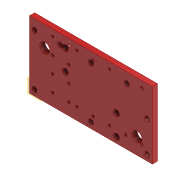
# Autodesk Inventor part: Motor mount to inside wall adapter
Saved by Autodesk Inventor 2020 (Build 240168000, 168)
## iProperties
Created: 2020-03-03
Part Number: Motor mount to inside wall adapter
Material: Generic
Document SubType Name: Modeling
Designer: ball
Density: 1 g/cm^3
Appearance: Default
Author: ball
Autodesk Inventor part; units mm, degrees
ref_plane "YZ Plane" through (0, 0, 0) normal (1, 0, 0) x (0, 1, 0)
ref_plane "XZ Plane" through (0, 0, 0) normal (0, 1, 0) x (-1, 0, 0)
ref_plane "XY Plane" through (0, 0, 0) normal (0, 0, 1) x (1, 0, 0)
ref_plane "Work Plane2" through (0, 0, 0) normal (0, 0, 1) x (1, 0, 0)
sketch "Sketch1" plane through (0, 0, 0) normal (0, 0, 1) x (1, 0, 0)
  line L0 (192, 96) -> (192, 48) construction
  line L1 (0, 96) -> (0, 48) construction
  line L2 (0, 0) -> (0, 48) construction
  line L3 (0, 0) -> (0, 96)
  line L4 (192, 96) -> (192, 0)
  circle A0 centre (184, 8) radius 2 construction
  circle A1 centre (8, 8) radius 2 construction
  circle A2 centre (8, 88) radius 2 construction
  circle A3 centre (184, 56) radius 2 construction
  arc A4 (98, 88) -> (94, 88) centre (96, 88) ccw construction
  arc A5 (94, 8) -> (98, 8) centre (96, 8) ccw construction
  circle A6 centre (184, 8) radius 2.2
  circle A7 centre (96, 8) radius 2.2
  circle A8 centre (8, 8) radius 2.2
  circle A9 centre (8, 88) radius 2.2
  circle A10 centre (96, 88) radius 2.2
  circle A11 centre (184, 56) radius 2.2
  circle A12 centre (152, 88) radius 2 construction
  circle A13 centre (152, 88) radius 2.2
  circle A14 centre (56, 88) radius 3.5 construction
  circle A15 centre (56, 56) radius 3.5 construction
  circle A16 centre (136, 8) radius 3.5 construction
  circle A17 centre (136, 40) radius 3.5 construction
  circle A18 centre (136, 8) radius 4.5
  circle A19 centre (136, 40) radius 4.5
  circle A20 centre (56, 88) radius 4.5
  circle A21 centre (56, 56) radius 4.5
  circle A22 centre (24, 72) radius 7.78 projected
  circle A23 centre (168, 24) radius 7.78 projected
  line L5 (0, 96) -> (0, 103.6708)
  line L6 (0, 103.6708) -> (192, 103.6708)
  line L7 (192, 103.6708) -> (192, 96)
  line L8 (0, 0) -> (0, -1.2954)
  line L9 (0, -1.2954) -> (192, -1.2954)
  line L10 (192, -1.2954) -> (192, 0)
  dimension "d0" = 4.4
  dimension "d1" = 4.4
  dimension "d2" = 4.4
  dimension "d3" = 4.4
  dimension "d4" = 4.4
  dimension "d5" = 4.4
  dimension "d6" = 4.4
  dimension "d7" = 9
  dimension "d8" = 9
  dimension "d9" = 9
  dimension "d10" = 9
  constraints: 16 end point, 11 centre point, 11 coincident, 3 parallel, 1 point on line
  measures "d0" diameter of A6
  measures "d1" diameter of A7
  measures "d2" diameter of A8
  measures "d3" diameter of A9
  measures "d4" diameter of A10
  measures "d5" diameter of A11
  measures "d6" diameter of A13
  measures "d7" diameter of A18
  measures "d8" diameter of A19
  measures "d9" diameter of A20
  measures "d10" diameter of A21
extrude "Extrusion1" add sketch "Sketch1" along normal blind 8
sketch "Sketch2" plane through (0, 0, 8) normal (0, 0, 1) x (1, 0, 0)
  circle A0 centre (184, 8) radius 2.2 construction
  circle A1 centre (184, 8) radius 4.115 construction
  line L0 (184, 12.115) -> (187.5637, 10.0575)
  line L1 (187.5637, 10.0575) -> (187.5637, 5.9425)
  line L2 (187.5637, 5.9425) -> (184, 3.885)
  line L3 (184, 3.885) -> (180.4363, 5.9425)
  line L4 (180.4363, 5.9425) -> (180.4363, 10.0575)
  line L5 (180.4363, 10.0575) -> (184, 12.115)
  circle A2 centre (96, 8) radius 2.2 construction
  circle A3 centre (96, 8) radius 4.115 construction
  circle A4 centre (8, 8) radius 2.2 construction
  circle A5 centre (8, 8) radius 4.115 construction
  circle A6 centre (8, 88) radius 2.2 construction
  circle A7 centre (8, 88) radius 4.115 construction
  circle A8 centre (96, 88) radius 2.2 construction
  circle A9 centre (96, 88) radius 4.115 construction
  circle A10 centre (184, 56) radius 2.2 construction
  circle A11 centre (184, 56) radius 4.115 construction
  line L6 (184, 60.115) -> (187.5637, 58.0575)
  line L7 (187.5637, 58.0575) -> (187.5637, 53.9425)
  line L8 (187.5637, 53.9425) -> (184, 51.885)
  line L9 (184, 51.885) -> (180.4363, 53.9425)
  line L10 (180.4363, 53.9425) -> (180.4363, 58.0575)
  line L11 (180.4363, 58.0575) -> (184, 60.115)
  line L12 (96, 92.115) -> (99.5637, 90.0575)
  line L13 (99.5637, 90.0575) -> (99.5637, 85.9425)
  line L14 (99.5637, 85.9425) -> (96, 83.885)
  line L15 (96, 83.885) -> (92.4363, 85.9425)
  line L16 (92.4363, 85.9425) -> (92.4363, 90.0575)
  line L17 (92.4363, 90.0575) -> (96, 92.115)
  line L18 (8, 92.115) -> (11.5637, 90.0575)
  line L19 (11.5637, 90.0575) -> (11.5637, 85.9425)
  line L20 (11.5637, 85.9425) -> (8, 83.885)
  line L21 (8, 83.885) -> (4.4363, 85.9425)
  line L22 (4.4363, 85.9425) -> (4.4363, 90.0575)
  line L23 (4.4363, 90.0575) -> (8, 92.115)
  line L24 (8, 12.115) -> (11.5637, 10.0575)
  line L25 (11.5637, 10.0575) -> (11.5637, 5.9425)
  line L26 (11.5637, 5.9425) -> (8, 3.885)
  line L27 (8, 3.885) -> (4.4363, 5.9425)
  line L28 (4.4363, 5.9425) -> (4.4363, 10.0575)
  line L29 (4.4363, 10.0575) -> (8, 12.115)
  line L30 (96, 12.115) -> (99.5637, 10.0575)
  line L31 (99.5637, 10.0575) -> (99.5637, 5.9425)
  line L32 (99.5637, 5.9425) -> (96, 3.885)
  line L33 (96, 3.885) -> (92.4363, 5.9425)
  line L34 (92.4363, 5.9425) -> (92.4363, 10.0575)
  line L35 (92.4363, 10.0575) -> (96, 12.115)
  circle A12 centre (152, 88) radius 2.2 construction
  circle A13 centre (152, 88) radius 4.115 construction
  line L36 (152, 92.115) -> (155.5637, 90.0575)
  line L37 (155.5637, 90.0575) -> (155.5637, 85.9425)
  line L38 (155.5637, 85.9425) -> (152, 83.885)
  line L39 (152, 83.885) -> (148.4363, 85.9425)
  line L40 (148.4363, 85.9425) -> (148.4363, 90.0575)
  line L41 (148.4363, 90.0575) -> (152, 92.115)
  point P0 (0, 0)
  dimension "d13" = 8.23
  dimension "d16" = 8.23
  dimension "d17" = 8.23
  dimension "d18" = 8.23
  dimension "d19" = 8.23
  dimension "d20" = 8.23
  dimension "d66" = 8.23
  constraints: 84 end point, 14 coincident, 7 vertical alignment, 105 other
extrude "Nut Well 4mm" cut sketch "Sketch2" against normal blind 5.5
sketch "Sketch3" plane through (0, 0, 0) normal (0, 0, -1) x (-1, 0, 0)
  circle A0 centre (-36.0247, 17.3171) radius 1.9304 construction
  circle A1 centre (-61.4247, 17.3171) radius 1.9304 construction
  circle A2 centre (-61.4247, 42.7171) radius 1.9304 construction
  circle A3 centre (-36.0247, 42.7171) radius 1.9304 construction
  circle A4 centre (-36.0247, 68.1171) radius 1.9304 construction
  circle A5 centre (-61.4247, 68.1171) radius 1.9304 construction
  circle A6 centre (-61.4247, 93.5171) radius 1.9304 construction
  circle A7 centre (-36.0247, 93.5171) radius 1.9304 construction
  circle A8 centre (-74.1247, 93.5171) radius 1.9304 construction
  circle A9 centre (-99.5247, 93.5171) radius 1.9304 construction
  circle A10 centre (-124.9247, 93.5171) radius 1.9304 construction
  circle A11 centre (-99.5247, 68.1171) radius 1.9304 construction
  circle A12 centre (-74.1247, 68.1171) radius 1.9304 construction
  circle A13 centre (-74.1247, 42.7171) radius 1.9304 construction
  circle A14 centre (-99.5247, 42.7171) radius 1.9304 construction
  circle A15 centre (-124.9247, 42.7171) radius 1.9304 construction
  line L0 (-192, -1.2954) -> (-192, 103.6708) construction
  line L1 (0, -1.2954) -> (-192, -1.2954) construction
  line L2 (0, 103.6708) -> (0, -1.2954) construction
  line L3 (-192, 103.6708) -> (0, 103.6708) construction
  circle A16 centre (-168, 24) radius 7.78 construction
  circle A17 centre (-56, 56) radius 4.5 construction
  circle A18 centre (-136, 40) radius 4.5 construction
  circle A19 centre (-184, 8) radius 2.2 construction
  circle A20 centre (-96, 8) radius 2.2 construction
  circle A21 centre (-8, 8) radius 2.2 construction
  circle A22 centre (-8, 88) radius 2.2 construction
  circle A23 centre (-96, 88) radius 2.2 construction
  circle A24 centre (-184, 56) radius 2.2 construction
  circle A25 centre (-152, 88) radius 2.2 construction
  circle A26 centre (-136, 8) radius 4.5 construction
  circle A27 centre (-56, 88) radius 4.5 construction
  circle A28 centre (-24, 72) radius 7.78 construction
  circle A29 centre (-124.9247, 68.1171) radius 1.9304 construction
  circle A30 centre (-150.3247, 68.1171) radius 1.9304 construction
  circle A31 centre (-175.7247, 68.1171) radius 1.9304 construction
  circle A32 centre (-150.3247, 42.7171) radius 1.9304 construction
  circle A33 centre (-175.7247, 42.7171) radius 1.9304 construction
  circle A34 centre (-175.7247, 17.3171) radius 1.9304 construction
  circle A35 centre (-150.3247, 17.3171) radius 1.9304 construction
  circle A36 centre (-124.9247, 17.3171) radius 1.9304 construction
  circle A37 centre (-99.5247, 17.3171) radius 1.9304 construction
  circle A38 centre (-74.1247, 17.3171) radius 1.9304 construction
  circle A39 centre (-175.7247, 93.5171) radius 1.9304 construction
  circle A40 centre (-150.3247, 93.5171) radius 1.9304 construction
  circle A41 centre (-36.0247, 17.3171) radius 1.9304
  circle A42 centre (-36.0247, 42.7171) radius 1.9304
  circle A43 centre (-36.0247, 68.1171) radius 1.9304
  circle A44 centre (-36.0247, 93.5171) radius 1.9304
  circle A45 centre (-61.4247, 68.1171) radius 1.9304
  circle A46 centre (-61.4247, 42.7171) radius 1.9304
  circle A47 centre (-61.4247, 17.3171) radius 1.9304
  circle A48 centre (-74.1247, 93.5171) radius 1.9304
  circle A49 centre (-74.1247, 17.3171) radius 1.9304
  circle A50 centre (-99.5247, 17.3171) radius 1.9304
  circle A51 centre (-124.9247, 17.3171) radius 1.9304
  circle A52 centre (-150.3247, 17.3171) radius 1.9304
  circle A53 centre (-175.7247, 17.3171) radius 1.9304
  circle A54 centre (-175.7247, 93.5171) radius 1.9304
  circle A55 centre (-124.9247, 93.5171) radius 1.9304
  circle A56 centre (-99.5247, 93.5171) radius 1.9304
  circle A57 centre (-56, 88) radius 3.5052 construction
  circle A58 centre (-61.4247, 93.5171) radius 1.9304
  point P0 (0, 0)
  dimension "SixClearanceHole" = 3.8608
  dimension "d26" = 3.8608
  dimension "d27" = 3.8608
  dimension "d28" = 3.8608
  dimension "d29" = 3.8608
  dimension "d30" = 3.8608
  dimension "d31" = 3.8608
  dimension "d32" = 3.8608
  dimension "d33" = 3.8608
  dimension "d34" = 3.8608
  dimension "d35" = 3.8608
  dimension "d36" = 3.8608
  dimension "d37" = 3.8608
  dimension "d38" = 3.8608
  dimension "d39" = 3.8608
  dimension "d40" = 3.8608
  dimension "d41" = 7.0104
  dimension "d42" = 3.8608
  constraints: 18 centre point, 18 coincident
  measures "SixClearanceHole" diameter of A41
  measures "d26" diameter of A42
  measures "d27" diameter of A43
  measures "d28" diameter of A44
  measures "d29" diameter of A45
  measures "d30" diameter of A46
  measures "d31" diameter of A47
  measures "d32" diameter of A48
  measures "d33" diameter of A49
  measures "d34" diameter of A50
  measures "d35" diameter of A51
  measures "d36" diameter of A52
  measures "d37" diameter of A53
  measures "d38" diameter of A54
  measures "d39" diameter of A55
  measures "d40" diameter of A56
  measures "d41" diameter of A57
  measures "d42" diameter of A58
extrude "Extrusion3" cut sketch "Sketch3" against normal through all
sketch "Sketch4" plane through (0, 0, 0) normal (0, 0, -1) x (-1, 0, 0)
  circle A0 centre (-36.0247, 17.3171) radius 1.9304 construction
  circle A1 centre (-36.0247, 17.3171) radius 4.6609 construction
  line L0 (-36.0247, 21.978) -> (-31.9883, 19.6475)
  line L1 (-31.9883, 19.6475) -> (-31.9883, 14.9866)
  line L2 (-31.9883, 14.9866) -> (-36.0247, 12.6562)
  line L3 (-36.0247, 12.6562) -> (-40.0612, 14.9866)
  line L4 (-40.0612, 14.9866) -> (-40.0612, 19.6475)
  line L5 (-40.0612, 19.6475) -> (-36.0247, 21.978)
  circle A2 centre (-36.0247, 42.7171) radius 1.9304 construction
  circle A3 centre (-36.0247, 68.1171) radius 1.9304 construction
  circle A4 centre (-36.0247, 93.5171) radius 1.9304 construction
  circle A5 centre (-74.1247, 93.5171) radius 1.9304 construction
  circle A6 centre (-124.9247, 93.5171) radius 1.9304 construction
  circle A7 centre (-175.7247, 93.5171) radius 1.9304 construction
  circle A8 centre (-184, 8) radius 2.2 construction
  circle A9 centre (-61.4247, 68.1171) radius 1.9304 construction
  circle A10 centre (-61.4247, 42.7171) radius 1.9304 construction
  circle A11 centre (-61.4247, 17.3171) radius 1.9304 construction
  circle A12 centre (-36.0247, 42.7171) radius 4.6609 construction
  line L6 (-36.0247, 47.378) -> (-31.9883, 45.0475)
  line L7 (-31.9883, 45.0475) -> (-31.9883, 40.3866)
  line L8 (-31.9883, 40.3866) -> (-36.0247, 38.0562)
  line L9 (-36.0247, 38.0562) -> (-40.0612, 40.3866)
  line L10 (-40.0612, 40.3866) -> (-40.0612, 45.0475)
  line L11 (-40.0612, 45.0475) -> (-36.0247, 47.378)
  circle A13 centre (-36.0247, 68.1171) radius 4.6609 construction
  line L12 (-36.0247, 72.778) -> (-31.9883, 70.4475)
  line L13 (-31.9883, 70.4475) -> (-31.9883, 65.7866)
  line L14 (-31.9883, 65.7866) -> (-36.0247, 63.4562)
  line L15 (-36.0247, 63.4562) -> (-40.0612, 65.7866)
  line L16 (-40.0612, 65.7866) -> (-40.0612, 70.4475)
  line L17 (-40.0612, 70.4475) -> (-36.0247, 72.778)
  circle A14 centre (-36.0247, 93.5171) radius 4.6609 construction
  line L18 (-36.0247, 98.178) -> (-31.9883, 95.8475)
  line L19 (-31.9883, 95.8475) -> (-31.9883, 91.1866)
  line L20 (-31.9883, 91.1866) -> (-36.0247, 88.8562)
  line L21 (-36.0247, 88.8562) -> (-40.0612, 91.1866)
  line L22 (-40.0612, 91.1866) -> (-40.0612, 95.8475)
  line L23 (-40.0612, 95.8475) -> (-36.0247, 98.178)
  circle A15 centre (-61.4247, 68.1171) radius 4.6609 construction
  line L24 (-61.4247, 72.778) -> (-57.3883, 70.4475)
  line L25 (-57.3883, 70.4475) -> (-57.3883, 65.7866)
  line L26 (-57.3883, 65.7866) -> (-61.4247, 63.4562)
  line L27 (-61.4247, 63.4562) -> (-65.4612, 65.7866)
  line L28 (-65.4612, 65.7866) -> (-65.4612, 70.4475)
  line L29 (-65.4612, 70.4475) -> (-61.4247, 72.778)
  circle A16 centre (-61.4247, 42.7171) radius 4.6609 construction
  line L30 (-61.4247, 47.378) -> (-57.3883, 45.0475)
  line L31 (-57.3883, 45.0475) -> (-57.3883, 40.3866)
  line L32 (-57.3883, 40.3866) -> (-61.4247, 38.0562)
  line L33 (-61.4247, 38.0562) -> (-65.4612, 40.3866)
  line L34 (-65.4612, 40.3866) -> (-65.4612, 45.0475)
  line L35 (-65.4612, 45.0475) -> (-61.4247, 47.378)
  circle A17 centre (-61.4247, 17.3171) radius 4.6609 construction
  line L36 (-61.4247, 21.978) -> (-57.3883, 19.6475)
  line L37 (-57.3883, 19.6475) -> (-57.3883, 14.9866)
  line L38 (-57.3883, 14.9866) -> (-61.4247, 12.6562)
  line L39 (-61.4247, 12.6562) -> (-65.4612, 14.9866)
  line L40 (-65.4612, 14.9866) -> (-65.4612, 19.6475)
  line L41 (-65.4612, 19.6475) -> (-61.4247, 21.978)
  circle A18 centre (-61.4247, 93.5171) radius 1.9304 construction
  circle A19 centre (-61.4247, 93.5171) radius 4.6609 construction
  circle A20 centre (-74.1247, 93.5171) radius 4.6609 construction
  circle A21 centre (-124.9247, 93.5171) radius 4.6609 construction
  circle A22 centre (-175.7247, 93.5171) radius 4.6609 construction
  line L42 (-61.4247, 98.178) -> (-57.3883, 95.8475)
  line L43 (-57.3883, 95.8475) -> (-57.3883, 91.1866)
  line L44 (-57.3883, 91.1866) -> (-61.4247, 88.8562)
  line L45 (-61.4247, 88.8562) -> (-65.4612, 91.1866)
  line L46 (-65.4612, 91.1866) -> (-65.4612, 95.8475)
  line L47 (-65.4612, 95.8475) -> (-61.4247, 98.178)
  line L48 (-74.1247, 98.178) -> (-70.0883, 95.8475)
  line L49 (-70.0883, 95.8475) -> (-70.0883, 91.1866)
  line L50 (-70.0883, 91.1866) -> (-74.1247, 88.8562)
  line L51 (-74.1247, 88.8562) -> (-78.1612, 91.1866)
  line L52 (-78.1612, 91.1866) -> (-78.1612, 95.8475)
  line L53 (-78.1612, 95.8475) -> (-74.1247, 98.178)
  line L54 (-124.9247, 98.178) -> (-120.8883, 95.8475)
  line L55 (-120.8883, 95.8475) -> (-120.8883, 91.1866)
  line L56 (-120.8883, 91.1866) -> (-124.9247, 88.8562)
  line L57 (-124.9247, 88.8562) -> (-128.9612, 91.1866)
  line L58 (-128.9612, 91.1866) -> (-128.9612, 95.8475)
  line L59 (-128.9612, 95.8475) -> (-124.9247, 98.178)
  line L60 (-175.7247, 98.178) -> (-171.6883, 95.8475)
  line L61 (-171.6883, 95.8475) -> (-171.6883, 91.1866)
  line L62 (-171.6883, 91.1866) -> (-175.7247, 88.8562)
  line L63 (-175.7247, 88.8562) -> (-179.7612, 91.1866)
  line L64 (-179.7612, 91.1866) -> (-179.7612, 95.8475)
  line L65 (-179.7612, 95.8475) -> (-175.7247, 98.178)
  point P0 (0, 0)
  point P1 (-99.5247, 93.5171)
  dimension "d45" = 9.3218
  dimension "d49" = 9.3218
  dimension "d50" = 9.3218
  dimension "d51" = 9.3218
  dimension "d52" = 9.3218
  dimension "d53" = 9.3218
  dimension "d73" = 9.3218
  dimension "d74" = 9.3218
  dimension "d76" = 9.3218
  dimension "d77" = 9.3218
  dimension "SixNutWell" = 9.3218
  constraints: 132 end point, 11 vertical alignment, 10 coincident, 165 other
extrude "Lift receiver nut wells thick plastic" cut sketch "Sketch4" against normal blind 6.7564
sketch "Sketch5" plane through (0, 0, 0) normal (0, 0, -1) x (-1, 0, 0)
  circle A0 centre (-74.1247, 17.3171) radius 1.9304 construction
  circle A1 centre (-74.1247, 17.3171) radius 4.6609 construction
  circle A2 centre (-99.5247, 17.3171) radius 1.9304 construction
  circle A3 centre (-99.5247, 17.3171) radius 4.6609 construction
  circle A4 centre (-124.9247, 17.3171) radius 1.9304 construction
  circle A5 centre (-124.9247, 17.3171) radius 4.6609 construction
  circle A6 centre (-150.3247, 17.3171) radius 1.9304 construction
  circle A7 centre (-150.3247, 17.3171) radius 4.6609 construction
  line L0 (-74.1247, 21.978) -> (-70.0883, 19.6475)
  line L1 (-70.0883, 19.6475) -> (-70.0883, 14.9866)
  line L2 (-70.0883, 14.9866) -> (-74.1247, 12.6562)
  line L3 (-74.1247, 12.6562) -> (-78.1612, 14.9866)
  line L4 (-78.1612, 14.9866) -> (-78.1612, 19.6475)
  line L5 (-78.1612, 19.6475) -> (-74.1247, 21.978)
  line L6 (-99.5247, 21.978) -> (-95.4883, 19.6475)
  line L7 (-95.4883, 19.6475) -> (-95.4883, 14.9866)
  line L8 (-95.4883, 14.9866) -> (-99.5247, 12.6562)
  line L9 (-99.5247, 12.6562) -> (-103.5612, 14.9866)
  line L10 (-103.5612, 14.9866) -> (-103.5612, 19.6475)
  line L11 (-103.5612, 19.6475) -> (-99.5247, 21.978)
  line L12 (-124.9247, 21.978) -> (-120.8883, 19.6475)
  line L13 (-120.8883, 19.6475) -> (-120.8883, 14.9866)
  line L14 (-120.8883, 14.9866) -> (-124.9247, 12.6562)
  line L15 (-124.9247, 12.6562) -> (-128.9612, 14.9866)
  line L16 (-128.9612, 14.9866) -> (-128.9612, 19.6475)
  line L17 (-128.9612, 19.6475) -> (-124.9247, 21.978)
  line L18 (-150.3247, 21.978) -> (-146.2883, 19.6475)
  line L19 (-146.2883, 19.6475) -> (-146.2883, 14.9866)
  line L20 (-146.2883, 14.9866) -> (-150.3247, 12.6562)
  line L21 (-150.3247, 12.6562) -> (-154.3612, 14.9866)
  line L22 (-154.3612, 14.9866) -> (-154.3612, 19.6475)
  line L23 (-154.3612, 19.6475) -> (-150.3247, 21.978)
  point P0 (0, 0)
  dimension "d78" = 9.3218
  dimension "d79" = 9.3218
  dimension "d80" = 9.3218
  dimension "d81" = 9.3218
  constraints: 48 end point, 9 coincident, 4 vertical alignment, 60 other
extrude "Lift receiver nut wells thin plastic" cut sketch "Sketch5" against normal blind 6.9088
sketch "Sketch6" plane through (0, 0, 0) normal (0, 0, -1) x (-1, 0, 0)
  line L0 (-24.7886, 9.4478) -> (-24.7886, 4.073)
  line L1 (-24.7886, 4.073) -> (-22.7434, 4.073)
  line L2 (-22.7434, 4.073) -> (-22.7434, 3.3518)
  line L3 (-22.7434, 3.3518) -> (-27.6439, 3.3518)
  line L4 (-27.6439, 3.3518) -> (-27.6439, 4.073)
  line L5 (-27.6439, 4.073) -> (-25.5988, 4.073)
  line L6 (-25.5988, 4.073) -> (-25.5988, 9.4478)
  line L7 (-25.5988, 9.4478) -> (-24.7886, 9.4478)
  spline S0 degree 2 poles (-32.5741, 4.0483) (-32.9199, 4.4534) (-33.3052, 5.639) (-33.3052, 6.3998) knots 0 0 0 1 2 2 2
  spline S1 degree 2 poles (-33.3052, 6.3998) (-33.3052, 7.1408) (-32.9298, 8.3412) (-32.5741, 8.7463) knots 0 0 0 1 2 2 2
  spline S2 degree 2 poles (-32.5741, 8.7463) (-32.1987, 9.1711) (-31.2057, 9.5762) (-30.608, 9.5762) knots 0 0 0 1 2 2 2
  spline S3 degree 2 poles (-30.608, 9.5762) (-29.9905, 9.5762) (-29.0024, 9.1563) (-28.6418, 8.7463) knots 0 0 0 1 2 2 2
  spline S4 degree 2 poles (-28.6418, 8.7463) (-28.2911, 8.3412) (-27.9156, 7.1507) (-27.9156, 6.3998) knots 0 0 0 1 2 2 2
  spline S5 degree 2 poles (-27.9156, 6.3998) (-27.9156, 5.6341) (-28.296, 4.4682) (-28.6468, 4.0483) knots 0 0 0 1 2 2 2
  spline S6 degree 2 poles (-28.6468, 4.0483) (-29.0024, 3.6432) (-29.9954, 3.2233) (-30.608, 3.2233) knots 0 0 0 1 2 2 2
  spline S7 degree 2 poles (-30.608, 3.2233) (-31.2304, 3.2233) (-32.2283, 3.6581) (-32.5741, 4.0483) knots 0 0 0 1 2 2 2
  spline S8 degree 2 poles (-32.4605, 6.3998) (-32.4605, 5.7971) (-32.1987, 4.8634) (-31.9615, 4.5571) knots 0 0 0 1 2 2 2
  spline S9 degree 2 poles (-31.9615, 4.5571) (-31.7195, 4.241) (-31.0377, 3.9248) (-30.6129, 3.9248) knots 0 0 0 1 2 2 2
  spline S10 degree 2 poles (-30.6129, 3.9248) (-30.1732, 3.9248) (-29.5113, 4.2311) (-29.2593, 4.5571) knots 0 0 0 1 2 2 2
  spline S11 degree 2 poles (-29.2593, 4.5571) (-29.0173, 4.8684) (-28.7604, 5.807) (-28.7604, 6.3998) knots 0 0 0 1 2 2 2
  spline S12 degree 2 poles (-28.7604, 6.3998) (-28.7604, 7.6002) (-29.7682, 8.8747) (-30.6129, 8.8747) knots 0 0 0 1 2 2 2
  spline S13 degree 2 poles (-30.6129, 8.8747) (-31.4576, 8.8747) (-32.4605, 7.6002) (-32.4605, 6.3998) knots 0 0 0 1 2 2 2
  spline S14 degree 2 poles (-38.0476, 5.1895) (-38.0476, 5.5847) (-37.7661, 6.296) (-37.5141, 6.543) knots 0 0 0 1 2 2 2
  spline S15 degree 2 poles (-37.5141, 6.543) (-37.198, 6.8543) (-36.3433, 7.1754) (-35.6913, 7.1754) knots 0 0 0 1 2 2 2
  line L8 (-35.6913, 7.1754) -> (-35.0046, 7.1754)
  line L9 (-35.0046, 7.1754) -> (-35.0046, 9.4478)
  line L10 (-35.0046, 9.4478) -> (-34.1944, 9.4478)
  line L11 (-34.1944, 9.4478) -> (-34.1944, 3.3518)
  line L12 (-34.1944, 3.3518) -> (-35.7258, 3.3518)
  spline S16 degree 2 poles (-35.7258, 3.3518) (-36.2692, 3.3518) (-37.03, 3.5296) (-37.3215, 3.7322) knots 0 0 0 1 2 2 2
  spline S17 degree 2 poles (-37.3215, 3.7322) (-37.6623, 3.9643) (-38.0476, 4.6806) (-38.0476, 5.1895) knots 0 0 0 1 2 2 2
  spline S18 degree 2 poles (-37.2029, 5.2142) (-37.2029, 4.898) (-36.9855, 4.4336) (-36.7632, 4.2854) knots 0 0 0 1 2 2 2
  spline S19 degree 2 poles (-36.7632, 4.2854) (-36.5706, 4.157) (-36.0568, 4.0533) (-35.6764, 4.0533) knots 0 0 0 1 2 2 2
  line L13 (-35.6764, 4.0533) -> (-35.0046, 4.0533)
  line L14 (-35.0046, 4.0533) -> (-35.0046, 6.4838)
  line L15 (-35.0046, 6.4838) -> (-35.5579, 6.4838)
  spline S20 degree 2 poles (-35.5579, 6.4838) (-36.0519, 6.4838) (-36.6595, 6.3257) (-36.8571, 6.1182) knots 0 0 0 1 2 2 2
  spline S21 degree 2 poles (-36.8571, 6.1182) (-37.0399, 5.9354) (-37.2029, 5.5056) (-37.2029, 5.2142) knots 0 0 0 1 2 2 2
  line L16 (-78.4457, 43.6737) -> (-78.4457, 38.2989)
  line L17 (-78.4457, 38.2989) -> (-76.4006, 38.2989)
  line L18 (-76.4006, 38.2989) -> (-76.4006, 37.5777)
  line L19 (-76.4006, 37.5777) -> (-81.3011, 37.5777)
  line L20 (-81.3011, 37.5777) -> (-81.3011, 38.2989)
  line L21 (-81.3011, 38.2989) -> (-79.2559, 38.2989)
  line L22 (-79.2559, 38.2989) -> (-79.2559, 43.6737)
  line L23 (-79.2559, 43.6737) -> (-78.4457, 43.6737)
  line L24 (-86.3448, 43.6737) -> (-85.5347, 43.6737)
  line L25 (-85.5347, 43.6737) -> (-85.5347, 40.6899)
  line L26 (-85.5347, 40.6899) -> (-82.7287, 40.6899)
  line L27 (-82.7287, 40.6899) -> (-82.7287, 43.6737)
  line L28 (-82.7287, 43.6737) -> (-81.9186, 43.6737)
  line L29 (-81.9186, 43.6737) -> (-81.9186, 37.5777)
  line L30 (-81.9186, 37.5777) -> (-82.7287, 37.5777)
  line L31 (-82.7287, 37.5777) -> (-82.7287, 39.9686)
  line L32 (-82.7287, 39.9686) -> (-85.5347, 39.9686)
  line L33 (-85.5347, 39.9686) -> (-85.5347, 37.5777)
  line L34 (-85.5347, 37.5777) -> (-86.3448, 37.5777)
  line L35 (-86.3448, 37.5777) -> (-86.3448, 43.6737)
  line L36 (-89.7041, 43.6737) -> (-87.3427, 43.6737)
  line L37 (-87.3427, 43.6737) -> (-87.3427, 43.0512)
  line L38 (-87.3427, 43.0512) -> (-88.1183, 43.0512)
  line L39 (-88.1183, 43.0512) -> (-88.1183, 38.2001)
  line L40 (-88.1183, 38.2001) -> (-87.3427, 38.2001)
  line L41 (-87.3427, 38.2001) -> (-87.3427, 37.5777)
  line L42 (-87.3427, 37.5777) -> (-89.7041, 37.5777)
  line L43 (-89.7041, 37.5777) -> (-89.7041, 38.2001)
  line L44 (-89.7041, 38.2001) -> (-88.9285, 38.2001)
  line L45 (-88.9285, 38.2001) -> (-88.9285, 43.0512)
  line L46 (-88.9285, 43.0512) -> (-89.7041, 43.0512)
  line L47 (-89.7041, 43.0512) -> (-89.7041, 43.6737)
  spline S22 degree 2 poles (-92.4063, 43.7824) (-91.7443, 43.7824) (-90.8156, 43.5057) (-90.4055, 43.3081) knots 0 0 0 1 2 2 2
  line L48 (-90.4055, 43.3081) -> (-90.4055, 42.2905)
  line L49 (-90.4055, 42.2905) -> (-90.4648, 42.2905)
  spline S23 degree 2 poles (-90.4648, 42.2905) (-90.865, 42.6659) (-91.8777, 43.0809) (-92.347, 43.0809) knots 0 0 0 1 2 2 2
  spline S24 degree 2 poles (-92.347, 43.0809) (-93.0188, 43.0809) (-93.7055, 42.5226) (-93.7055, 42.0632) knots 0 0 0 1 2 2 2
  spline S25 degree 2 poles (-93.7055, 42.0632) (-93.7055, 41.6977) (-93.3449, 41.2432) (-92.9546, 41.1296) knots 0 0 0 1 2 2 2
  spline S26 degree 2 poles (-92.9546, 41.1296) (-92.673, 41.0505) (-92.2037, 40.9418) (-91.853, 40.8529) knots 0 0 0 1 2 2 2
  spline S27 degree 2 poles (-91.853, 40.8529) (-91.5368, 40.7689) (-91.0379, 40.517) (-90.8452, 40.3144) knots 0 0 0 1 2 2 2
  spline S28 degree 2 poles (-90.8452, 40.3144) (-90.6575, 40.1119) (-90.45, 39.5685) (-90.45, 39.2128) knots 0 0 0 1 2 2 2
  spline S29 degree 2 poles (-90.45, 39.2128) (-90.45, 38.4718) (-91.606, 37.469) (-92.5001, 37.469) knots 0 0 0 1 2 2 2
  spline S30 degree 2 poles (-92.5001, 37.469) (-93.0139, 37.469) (-93.9229, 37.6715) (-94.3131, 37.8642) knots 0 0 0 1 2 2 2
  line L50 (-94.3131, 37.8642) -> (-94.3131, 38.8324)
  line L51 (-94.3131, 38.8324) -> (-94.2538, 38.8324)
  spline S31 degree 2 poles (-94.2538, 38.8324) (-93.9624, 38.5657) (-93.0534, 38.1705) (-92.5545, 38.1705) knots 0 0 0 1 2 2 2
  spline S32 degree 2 poles (-92.5545, 38.1705) (-91.9913, 38.1705) (-91.2948, 38.6991) (-91.2948, 39.1288) knots 0 0 0 1 2 2 2
  spline S33 degree 2 poles (-91.2948, 39.1288) (-91.2948, 39.5142) (-91.7048, 39.9736) (-92.0901, 40.0773) knots 0 0 0 1 2 2 2
  spline S34 degree 2 poles (-92.0901, 40.0773) (-92.347, 40.1465) (-93.0929, 40.3243) (-93.3399, 40.3984) knots 0 0 0 1 2 2 2
  spline S35 degree 2 poles (-93.3399, 40.3984) (-93.9673, 40.5911) (-94.5502, 41.3667) (-94.5502, 41.9348) knots 0 0 0 1 2 2 2
  spline S36 degree 2 poles (-94.5502, 41.9348) (-94.5502, 42.2954) (-94.2588, 42.987) (-93.997, 43.2291) knots 0 0 0 1 2 2 2
  spline S37 degree 2 poles (-93.997, 43.2291) (-93.7055, 43.4958) (-92.9645, 43.7824) (-92.4063, 43.7824) knots 0 0 0 1 2 2 2
  spline S38 degree 2 poles (-99.6928, 43.7824) (-99.0308, 43.7824) (-98.1021, 43.5057) (-97.6921, 43.3081) knots 0 0 0 1 2 2 2
  line L52 (-97.6921, 43.3081) -> (-97.6921, 42.2905)
  line L53 (-97.6921, 42.2905) -> (-97.7514, 42.2905)
  spline S39 degree 2 poles (-97.7514, 42.2905) (-98.1515, 42.6659) (-99.1642, 43.0809) (-99.6335, 43.0809) knots 0 0 0 1 2 2 2
  spline S40 degree 2 poles (-99.6335, 43.0809) (-100.3054, 43.0809) (-100.992, 42.5226) (-100.992, 42.0632) knots 0 0 0 1 2 2 2
  spline S41 degree 2 poles (-100.992, 42.0632) (-100.992, 41.6977) (-100.6314, 41.2432) (-100.2412, 41.1296) knots 0 0 0 1 2 2 2
  spline S42 degree 2 poles (-100.2412, 41.1296) (-99.9596, 41.0505) (-99.4903, 40.9418) (-99.1395, 40.8529) knots 0 0 0 1 2 2 2
  spline S43 degree 2 poles (-99.1395, 40.8529) (-98.8234, 40.7689) (-98.3244, 40.517) (-98.1318, 40.3144) knots 0 0 0 1 2 2 2
  spline S44 degree 2 poles (-98.1318, 40.3144) (-97.944, 40.1119) (-97.7366, 39.5685) (-97.7366, 39.2128) knots 0 0 0 1 2 2 2
  spline S45 degree 2 poles (-97.7366, 39.2128) (-97.7366, 38.4718) (-98.8925, 37.469) (-99.7867, 37.469) knots 0 0 0 1 2 2 2
  spline S46 degree 2 poles (-99.7867, 37.469) (-100.3004, 37.469) (-101.2094, 37.6715) (-101.5997, 37.8642) knots 0 0 0 1 2 2 2
  line L54 (-101.5997, 37.8642) -> (-101.5997, 38.8324)
  line L55 (-101.5997, 38.8324) -> (-101.5404, 38.8324)
  spline S47 degree 2 poles (-101.5404, 38.8324) (-101.2489, 38.5657) (-100.34, 38.1705) (-99.841, 38.1705) knots 0 0 0 1 2 2 2
  spline S48 degree 2 poles (-99.841, 38.1705) (-99.2778, 38.1705) (-98.5813, 38.6991) (-98.5813, 39.1288) knots 0 0 0 1 2 2 2
  spline S49 degree 2 poles (-98.5813, 39.1288) (-98.5813, 39.5142) (-98.9913, 39.9736) (-99.3766, 40.0773) knots 0 0 0 1 2 2 2
  spline S50 degree 2 poles (-99.3766, 40.0773) (-99.6335, 40.1465) (-100.3795, 40.3243) (-100.6265, 40.3984) knots 0 0 0 1 2 2 2
  spline S51 degree 2 poles (-100.6265, 40.3984) (-101.2539, 40.5911) (-101.8368, 41.3667) (-101.8368, 41.9348) knots 0 0 0 1 2 2 2
  spline S52 degree 2 poles (-101.8368, 41.9348) (-101.8368, 42.2954) (-101.5453, 42.987) (-101.2835, 43.2291) knots 0 0 0 1 2 2 2
  spline S53 degree 2 poles (-101.2835, 43.2291) (-100.992, 43.4958) (-100.251, 43.7824) (-99.6928, 43.7824) knots 0 0 0 1 2 2 2
  line L56 (-104.786, 43.6737) -> (-102.4246, 43.6737)
  line L57 (-102.4246, 43.6737) -> (-102.4246, 43.0512)
  line L58 (-102.4246, 43.0512) -> (-103.2002, 43.0512)
  line L59 (-103.2002, 43.0512) -> (-103.2002, 38.2001)
  line L60 (-103.2002, 38.2001) -> (-102.4246, 38.2001)
  line L61 (-102.4246, 38.2001) -> (-102.4246, 37.5777)
  line L62 (-102.4246, 37.5777) -> (-104.786, 37.5777)
  line L63 (-104.786, 37.5777) -> (-104.786, 38.2001)
  line L64 (-104.786, 38.2001) -> (-104.0104, 38.2001)
  line L65 (-104.0104, 38.2001) -> (-104.0104, 43.0512)
  line L66 (-104.0104, 43.0512) -> (-104.786, 43.0512)
  line L67 (-104.786, 43.0512) -> (-104.786, 43.6737)
  spline S54 degree 2 poles (-110.5955, 40.6306) (-110.5955, 41.4655) (-109.9187, 42.8092) (-109.3506, 43.1846) knots 0 0 0 1 2 2 2
  spline S55 degree 2 poles (-109.3506, 43.1846) (-108.8862, 43.4761) (-107.9328, 43.6737) (-107.1918, 43.6737) knots 0 0 0 1 2 2 2
  line L68 (-107.1918, 43.6737) -> (-105.7888, 43.6737)
  line L69 (-105.7888, 43.6737) -> (-105.7888, 37.5777)
  line L70 (-105.7888, 37.5777) -> (-107.177, 37.5777)
  spline S56 degree 2 poles (-107.177, 37.5777) (-108.0365, 37.5777) (-109.0146, 37.8346) (-109.3605, 38.0618) knots 0 0 0 1 2 2 2
  spline S57 degree 2 poles (-109.3605, 38.0618) (-109.9483, 38.4521) (-110.5955, 39.7414) (-110.5955, 40.6306) knots 0 0 0 1 2 2 2
  spline S58 degree 2 poles (-109.7507, 40.6207) (-109.7507, 39.9192) (-109.2864, 38.9263) (-108.8269, 38.6447) knots 0 0 0 1 2 2 2
  spline S59 degree 2 poles (-108.8269, 38.6447) (-108.5009, 38.4521) (-107.7648, 38.2792) (-107.2165, 38.2792) knots 0 0 0 1 2 2 2
  line L71 (-107.2165, 38.2792) -> (-106.599, 38.2792)
  line L72 (-106.599, 38.2792) -> (-106.599, 42.9722)
  line L73 (-106.599, 42.9722) -> (-107.2165, 42.9722)
  spline S60 degree 2 poles (-107.2165, 42.9722) (-107.7549, 42.9722) (-108.57, 42.7993) (-108.901, 42.5671) knots 0 0 0 1 2 2 2
  spline S61 degree 2 poles (-108.901, 42.5671) (-109.3259, 42.2806) (-109.7507, 41.3321) (-109.7507, 40.6207) knots 0 0 0 1 2 2 2
  line L74 (-111.4748, 43.6737) -> (-111.4748, 37.5777)
  line L75 (-111.4748, 37.5777) -> (-115.2885, 37.5777)
  line L76 (-115.2885, 37.5777) -> (-115.2885, 38.2989)
  line L77 (-115.2885, 38.2989) -> (-112.285, 38.2989)
  line L78 (-112.285, 38.2989) -> (-112.285, 39.9686)
  line L79 (-112.285, 39.9686) -> (-115.0859, 39.9686)
  line L80 (-115.0859, 39.9686) -> (-115.0859, 40.6899)
  line L81 (-115.0859, 40.6899) -> (-112.285, 40.6899)
  line L82 (-112.285, 40.6899) -> (-112.285, 42.9524)
  line L83 (-112.285, 42.9524) -> (-115.2885, 42.9524)
  line L84 (-115.2885, 42.9524) -> (-115.2885, 43.6737)
  line L85 (-115.2885, 43.6737) -> (-111.4748, 43.6737)
  line L86 (-78.0467, 54.6668) -> (-78.0467, 49.292)
  line L87 (-78.0467, 49.292) -> (-76.0015, 49.292)
  line L88 (-76.0015, 49.292) -> (-76.0015, 48.5708)
  line L89 (-76.0015, 48.5708) -> (-80.902, 48.5708)
  line L90 (-80.902, 48.5708) -> (-80.902, 49.292)
  line L91 (-80.902, 49.292) -> (-78.8568, 49.292)
  line L92 (-78.8568, 49.292) -> (-78.8568, 54.6668)
  line L93 (-78.8568, 54.6668) -> (-78.0467, 54.6668)
  spline S62 degree 2 poles (-85.8322, 49.2673) (-86.178, 49.6724) (-86.5633, 50.858) (-86.5633, 51.6188) knots 0 0 0 1 2 2 2
  spline S63 degree 2 poles (-86.5633, 51.6188) (-86.5633, 52.3598) (-86.1879, 53.5602) (-85.8322, 53.9653) knots 0 0 0 1 2 2 2
  spline S64 degree 2 poles (-85.8322, 53.9653) (-85.4567, 54.3901) (-84.4638, 54.7952) (-83.866, 54.7952) knots 0 0 0 1 2 2 2
  spline S65 degree 2 poles (-83.866, 54.7952) (-83.2485, 54.7952) (-82.2605, 54.3753) (-81.8999, 53.9653) knots 0 0 0 1 2 2 2
  spline S66 degree 2 poles (-81.8999, 53.9653) (-81.5492, 53.5602) (-81.1737, 52.3696) (-81.1737, 51.6188) knots 0 0 0 1 2 2 2
  spline S67 degree 2 poles (-81.1737, 51.6188) (-81.1737, 50.8531) (-81.5541, 49.6872) (-81.9048, 49.2673) knots 0 0 0 1 2 2 2
  spline S68 degree 2 poles (-81.9048, 49.2673) (-82.2605, 48.8622) (-83.2535, 48.4423) (-83.866, 48.4423) knots 0 0 0 1 2 2 2
  spline S69 degree 2 poles (-83.866, 48.4423) (-84.4885, 48.4423) (-85.4864, 48.877) (-85.8322, 49.2673) knots 0 0 0 1 2 2 2
  spline S70 degree 2 poles (-85.7185, 51.6188) (-85.7185, 51.0161) (-85.4567, 50.0824) (-85.2196, 49.7761) knots 0 0 0 1 2 2 2
  spline S71 degree 2 poles (-85.2196, 49.7761) (-84.9775, 49.46) (-84.2958, 49.1438) (-83.871, 49.1438) knots 0 0 0 1 2 2 2
  spline S72 degree 2 poles (-83.871, 49.1438) (-83.4313, 49.1438) (-82.7693, 49.4501) (-82.5174, 49.7761) knots 0 0 0 1 2 2 2
  spline S73 degree 2 poles (-82.5174, 49.7761) (-82.2753, 50.0874) (-82.0185, 51.026) (-82.0185, 51.6188) knots 0 0 0 1 2 2 2
  spline S74 degree 2 poles (-82.0185, 51.6188) (-82.0185, 52.8192) (-83.0262, 54.0937) (-83.871, 54.0937) knots 0 0 0 1 2 2 2
  spline S75 degree 2 poles (-83.871, 54.0937) (-84.7157, 54.0937) (-85.7185, 52.8192) (-85.7185, 51.6188) knots 0 0 0 1 2 2 2
  line L94 (-95.2973, 54.6668) -> (-94.4871, 54.6668)
  line L95 (-94.4871, 54.6668) -> (-94.4871, 49.4155)
  line L96 (-94.4871, 49.4155) -> (-92.8964, 52.9871)
  line L97 (-92.8964, 52.9871) -> (-92.4024, 52.9871)
  line L98 (-92.4024, 52.9871) -> (-90.8265, 49.4155)
  line L99 (-90.8265, 49.4155) -> (-90.8265, 54.6668)
  line L100 (-90.8265, 54.6668) -> (-90.0707, 54.6668)
  line L101 (-90.0707, 54.6668) -> (-90.0707, 48.5708)
  line L102 (-90.0707, 48.5708) -> (-91.1773, 48.5708)
  line L103 (-91.1773, 48.5708) -> (-92.6988, 51.9646)
  line L104 (-92.6988, 51.9646) -> (-94.1709, 48.5708)
  line L105 (-94.1709, 48.5708) -> (-95.2973, 48.5708)
  line L106 (-95.2973, 48.5708) -> (-95.2973, 54.6668)
  spline S76 degree 2 poles (-100.8449, 49.2673) (-101.1907, 49.6724) (-101.5761, 50.858) (-101.5761, 51.6188) knots 0 0 0 1 2 2 2
  spline S77 degree 2 poles (-101.5761, 51.6188) (-101.5761, 52.3598) (-101.2006, 53.5602) (-100.8449, 53.9653) knots 0 0 0 1 2 2 2
  spline S78 degree 2 poles (-100.8449, 53.9653) (-100.4695, 54.3901) (-99.4765, 54.7952) (-98.8788, 54.7952) knots 0 0 0 1 2 2 2
  spline S79 degree 2 poles (-98.8788, 54.7952) (-98.2613, 54.7952) (-97.2733, 54.3753) (-96.9127, 53.9653) knots 0 0 0 1 2 2 2
  spline S80 degree 2 poles (-96.9127, 53.9653) (-96.5619, 53.5602) (-96.1865, 52.3696) (-96.1865, 51.6188) knots 0 0 0 1 2 2 2
  spline S81 degree 2 poles (-96.1865, 51.6188) (-96.1865, 50.8531) (-96.5669, 49.6872) (-96.9176, 49.2673) knots 0 0 0 1 2 2 2
  spline S82 degree 2 poles (-96.9176, 49.2673) (-97.2733, 48.8622) (-98.2662, 48.4423) (-98.8788, 48.4423) knots 0 0 0 1 2 2 2
  spline S83 degree 2 poles (-98.8788, 48.4423) (-99.5012, 48.4423) (-100.4991, 48.877) (-100.8449, 49.2673) knots 0 0 0 1 2 2 2
  spline S84 degree 2 poles (-100.7313, 51.6188) (-100.7313, 51.0161) (-100.4695, 50.0824) (-100.2324, 49.7761) knots 0 0 0 1 2 2 2
  spline S85 degree 2 poles (-100.2324, 49.7761) (-99.9903, 49.46) (-99.3086, 49.1438) (-98.8837, 49.1438) knots 0 0 0 1 2 2 2
  spline S86 degree 2 poles (-98.8837, 49.1438) (-98.4441, 49.1438) (-97.7821, 49.4501) (-97.5302, 49.7761) knots 0 0 0 1 2 2 2
  spline S87 degree 2 poles (-97.5302, 49.7761) (-97.2881, 50.0874) (-97.0312, 51.026) (-97.0312, 51.6188) knots 0 0 0 1 2 2 2
  spline S88 degree 2 poles (-97.0312, 51.6188) (-97.0312, 52.8192) (-98.039, 54.0937) (-98.8837, 54.0937) knots 0 0 0 1 2 2 2
  spline S89 degree 2 poles (-98.8837, 54.0937) (-99.7285, 54.0937) (-100.7313, 52.8192) (-100.7313, 51.6188) knots 0 0 0 1 2 2 2
  line L107 (-103.888, 54.6668) -> (-103.888, 49.292)
  line L108 (-103.888, 49.292) -> (-101.8428, 49.292)
  line L109 (-101.8428, 49.292) -> (-101.8428, 48.5708)
  line L110 (-101.8428, 48.5708) -> (-106.7433, 48.5708)
  line L111 (-106.7433, 48.5708) -> (-106.7433, 49.292)
  line L112 (-106.7433, 49.292) -> (-104.6982, 49.292)
  line L113 (-104.6982, 49.292) -> (-104.6982, 54.6668)
  line L114 (-104.6982, 54.6668) -> (-103.888, 54.6668)
  spline S90 degree 2 poles (-111.6735, 49.2673) (-112.0193, 49.6724) (-112.4046, 50.858) (-112.4046, 51.6188) knots 0 0 0 1 2 2 2
  spline S91 degree 2 poles (-112.4046, 51.6188) (-112.4046, 52.3598) (-112.0292, 53.5602) (-111.6735, 53.9653) knots 0 0 0 1 2 2 2
  spline S92 degree 2 poles (-111.6735, 53.9653) (-111.298, 54.3901) (-110.3051, 54.7952) (-109.7073, 54.7952) knots 0 0 0 1 2 2 2
  spline S93 degree 2 poles (-109.7073, 54.7952) (-109.0898, 54.7952) (-108.1018, 54.3753) (-107.7412, 53.9653) knots 0 0 0 1 2 2 2
  spline S94 degree 2 poles (-107.7412, 53.9653) (-107.3905, 53.5602) (-107.015, 52.3696) (-107.015, 51.6188) knots 0 0 0 1 2 2 2
  spline S95 degree 2 poles (-107.015, 51.6188) (-107.015, 50.8531) (-107.3954, 49.6872) (-107.7462, 49.2673) knots 0 0 0 1 2 2 2
  spline S96 degree 2 poles (-107.7462, 49.2673) (-108.1018, 48.8622) (-109.0948, 48.4423) (-109.7073, 48.4423) knots 0 0 0 1 2 2 2
  spline S97 degree 2 poles (-109.7073, 48.4423) (-110.3298, 48.4423) (-111.3277, 48.877) (-111.6735, 49.2673) knots 0 0 0 1 2 2 2
  spline S98 degree 2 poles (-111.5599, 51.6188) (-111.5599, 51.0161) (-111.298, 50.0824) (-111.0609, 49.7761) knots 0 0 0 1 2 2 2
  spline S99 degree 2 poles (-111.0609, 49.7761) (-110.8189, 49.46) (-110.1371, 49.1438) (-109.7123, 49.1438) knots 0 0 0 1 2 2 2
  spline S100 degree 2 poles (-109.7123, 49.1438) (-109.2726, 49.1438) (-108.6107, 49.4501) (-108.3587, 49.7761) knots 0 0 0 1 2 2 2
  spline S101 degree 2 poles (-108.3587, 49.7761) (-108.1167, 50.0874) (-107.8598, 51.026) (-107.8598, 51.6188) knots 0 0 0 1 2 2 2
  spline S102 degree 2 poles (-107.8598, 51.6188) (-107.8598, 52.8192) (-108.8675, 54.0937) (-109.7123, 54.0937) knots 0 0 0 1 2 2 2
  spline S103 degree 2 poles (-109.7123, 54.0937) (-110.557, 54.0937) (-111.5599, 52.8192) (-111.5599, 51.6188) knots 0 0 0 1 2 2 2
  line L115 (-118.0115, 54.6668) -> (-116.9593, 54.6668)
  line L116 (-116.9593, 54.6668) -> (-115.0327, 52.2412)
  line L117 (-115.0327, 52.2412) -> (-114.104, 52.2412)
  line L118 (-114.104, 52.2412) -> (-114.104, 54.6668)
  line L119 (-114.104, 54.6668) -> (-113.2938, 54.6668)
  line L120 (-113.2938, 54.6668) -> (-113.2938, 48.5708)
  line L121 (-113.2938, 48.5708) -> (-114.8647, 48.5708)
  spline S104 degree 2 poles (-114.8647, 48.5708) (-115.3884, 48.5708) (-116.0948, 48.6844) (-116.4159, 48.8919) knots 0 0 0 1 2 2 2
  spline S105 degree 2 poles (-116.4159, 48.8919) (-116.737, 49.0993) (-117.1075, 49.7465) (-117.1075, 50.2257) knots 0 0 0 1 2 2 2
  spline S106 degree 2 poles (-117.1075, 50.2257) (-117.1075, 50.8926) (-116.4258, 51.7966) (-115.8429, 52.014) knots 0 0 0 1 2 2 2
  line L122 (-115.8429, 52.014) -> (-118.0115, 54.6668)
  spline S107 degree 2 poles (-116.2628, 50.2899) (-116.2628, 50.0231) (-116.075, 49.6131) (-115.8774, 49.4797) knots 0 0 0 1 2 2 2
  spline S108 degree 2 poles (-115.8774, 49.4797) (-115.7045, 49.3661) (-115.2451, 49.2722) (-114.9092, 49.2722) knots 0 0 0 1 2 2 2
  line L123 (-114.9092, 49.2722) -> (-114.104, 49.2722)
  line L124 (-114.104, 49.2722) -> (-114.104, 51.5644)
  line L125 (-114.104, 51.5644) -> (-114.8153, 51.5644)
  spline S109 degree 2 poles (-114.8153, 51.5644) (-115.1661, 51.5644) (-115.7243, 51.4409) (-115.917, 51.2483) knots 0 0 0 1 2 2 2
  spline S110 degree 2 poles (-115.917, 51.2483) (-116.0948, 51.0803) (-116.2628, 50.6061) (-116.2628, 50.2899) knots 0 0 0 1 2 2 2
  line L126 (-148.0711, 72.9823) -> (-144.539, 72.9823)
  line L127 (-144.539, 72.9823) -> (-144.539, 66.8863)
  line L128 (-144.539, 66.8863) -> (-145.3492, 66.8863)
  line L129 (-145.3492, 66.8863) -> (-145.3492, 72.261)
  line L130 (-145.3492, 72.261) -> (-148.0711, 72.261)
  line L131 (-148.0711, 72.261) -> (-148.0711, 72.9823)
  line L132 (-148.7084, 72.9823) -> (-148.7084, 66.8863)
  line L133 (-148.7084, 66.8863) -> (-152.5221, 66.8863)
  line L134 (-152.5221, 66.8863) -> (-152.5221, 67.6075)
  line L135 (-152.5221, 67.6075) -> (-149.5185, 67.6075)
  line L136 (-149.5185, 67.6075) -> (-149.5185, 69.2772)
  line L137 (-149.5185, 69.2772) -> (-152.3195, 69.2772)
  line L138 (-152.3195, 69.2772) -> (-152.3195, 69.9985)
  line L139 (-152.3195, 69.9985) -> (-149.5185, 69.9985)
  line L140 (-149.5185, 69.9985) -> (-149.5185, 72.261)
  line L141 (-149.5185, 72.261) -> (-152.5221, 72.261)
  line L142 (-152.5221, 72.261) -> (-152.5221, 72.9823)
  line L143 (-152.5221, 72.9823) -> (-148.7084, 72.9823)
  line L144 (-157.057, 67.6075) -> (-154.2215, 67.6075)
  line L145 (-154.2215, 67.6075) -> (-154.2215, 69.3266)
  line L146 (-154.2215, 69.3266) -> (-156.9385, 69.3266)
  line L147 (-156.9385, 69.3266) -> (-156.9385, 70.0479)
  line L148 (-156.9385, 70.0479) -> (-154.2215, 70.0479)
  line L149 (-154.2215, 70.0479) -> (-154.2215, 72.9823)
  line L150 (-154.2215, 72.9823) -> (-153.4113, 72.9823)
  line L151 (-153.4113, 72.9823) -> (-153.4113, 66.8863)
  line L152 (-153.4113, 66.8863) -> (-157.057, 66.8863)
  line L153 (-157.057, 66.8863) -> (-157.057, 67.6075)
  line L154 (-159.206, 72.9823) -> (-159.206, 67.6075)
  line L155 (-159.206, 67.6075) -> (-157.1608, 67.6075)
  line L156 (-157.1608, 67.6075) -> (-157.1608, 66.8863)
  line L157 (-157.1608, 66.8863) -> (-162.0613, 66.8863)
  line L158 (-162.0613, 66.8863) -> (-162.0613, 67.6075)
  line L159 (-162.0613, 67.6075) -> (-160.0161, 67.6075)
  line L160 (-160.0161, 67.6075) -> (-160.0161, 72.9823)
  line L161 (-160.0161, 72.9823) -> (-159.206, 72.9823)
  spline S111 degree 2 poles (-166.9964, 73.091) (-166.3344, 73.091) (-165.4057, 72.8143) (-164.9957, 72.6167) knots 0 0 0 1 2 2 2
  line L162 (-164.9957, 72.6167) -> (-164.9957, 71.5991)
  line L163 (-164.9957, 71.5991) -> (-165.0549, 71.5991)
  spline S112 degree 2 poles (-165.0549, 71.5991) (-165.4551, 71.9745) (-166.4678, 72.3895) (-166.9371, 72.3895) knots 0 0 0 1 2 2 2
  spline S113 degree 2 poles (-166.9371, 72.3895) (-167.6089, 72.3895) (-168.2956, 71.8312) (-168.2956, 71.3718) knots 0 0 0 1 2 2 2
  spline S114 degree 2 poles (-168.2956, 71.3718) (-168.2956, 71.0063) (-167.935, 70.5518) (-167.5447, 70.4382) knots 0 0 0 1 2 2 2
  spline S115 degree 2 poles (-167.5447, 70.4382) (-167.2631, 70.3591) (-166.7938, 70.2504) (-166.4431, 70.1615) knots 0 0 0 1 2 2 2
  spline S116 degree 2 poles (-166.4431, 70.1615) (-166.1269, 70.0775) (-165.628, 69.8256) (-165.4353, 69.6231) knots 0 0 0 1 2 2 2
  spline S117 degree 2 poles (-165.4353, 69.6231) (-165.2476, 69.4205) (-165.0401, 68.8771) (-165.0401, 68.5214) knots 0 0 0 1 2 2 2
  spline S118 degree 2 poles (-165.0401, 68.5214) (-165.0401, 67.7804) (-166.1961, 66.7776) (-167.0902, 66.7776) knots 0 0 0 1 2 2 2
  spline S119 degree 2 poles (-167.0902, 66.7776) (-167.604, 66.7776) (-168.513, 66.9801) (-168.9032, 67.1728) knots 0 0 0 1 2 2 2
  line L164 (-168.9032, 67.1728) -> (-168.9032, 68.141)
  line L165 (-168.9032, 68.141) -> (-168.844, 68.141)
  spline S120 degree 2 poles (-168.844, 68.141) (-168.5525, 67.8743) (-167.6435, 67.4791) (-167.1446, 67.4791) knots 0 0 0 1 2 2 2
  spline S121 degree 2 poles (-167.1446, 67.4791) (-166.5814, 67.4791) (-165.8849, 68.0077) (-165.8849, 68.4374) knots 0 0 0 1 2 2 2
  spline S122 degree 2 poles (-165.8849, 68.4374) (-165.8849, 68.8228) (-166.2949, 69.2822) (-166.6802, 69.3859) knots 0 0 0 1 2 2 2
  spline S123 degree 2 poles (-166.6802, 69.3859) (-166.9371, 69.4551) (-167.683, 69.6329) (-167.93, 69.707) knots 0 0 0 1 2 2 2
  spline S124 degree 2 poles (-167.93, 69.707) (-168.5574, 69.8997) (-169.1404, 70.6753) (-169.1404, 71.2434) knots 0 0 0 1 2 2 2
  spline S125 degree 2 poles (-169.1404, 71.2434) (-169.1404, 71.604) (-168.8489, 72.2956) (-168.5871, 72.5377) knots 0 0 0 1 2 2 2
  spline S126 degree 2 poles (-168.5871, 72.5377) (-168.2956, 72.8044) (-167.5546, 73.091) (-166.9964, 73.091) knots 0 0 0 1 2 2 2
  line L166 (-172.0896, 72.9823) -> (-169.7282, 72.9823)
  line L167 (-169.7282, 72.9823) -> (-169.7282, 72.3598)
  line L168 (-169.7282, 72.3598) -> (-170.5038, 72.3598)
  line L169 (-170.5038, 72.3598) -> (-170.5038, 67.5087)
  line L170 (-170.5038, 67.5087) -> (-169.7282, 67.5087)
  line L171 (-169.7282, 67.5087) -> (-169.7282, 66.8863)
  line L172 (-169.7282, 66.8863) -> (-172.0896, 66.8863)
  line L173 (-172.0896, 66.8863) -> (-172.0896, 67.5087)
  line L174 (-172.0896, 67.5087) -> (-171.314, 67.5087)
  line L175 (-171.314, 67.5087) -> (-171.314, 72.3598)
  line L176 (-171.314, 72.3598) -> (-172.0896, 72.3598)
  line L177 (-172.0896, 72.3598) -> (-172.0896, 72.9823)
  spline S127 degree 2 poles (-177.899, 69.9392) (-177.899, 70.7741) (-177.2222, 72.1178) (-176.6541, 72.4932) knots 0 0 0 1 2 2 2
  spline S128 degree 2 poles (-176.6541, 72.4932) (-176.1898, 72.7847) (-175.2364, 72.9823) (-174.4954, 72.9823) knots 0 0 0 1 2 2 2
  line L178 (-174.4954, 72.9823) -> (-173.0924, 72.9823)
  line L179 (-173.0924, 72.9823) -> (-173.0924, 66.8863)
  line L180 (-173.0924, 66.8863) -> (-174.4805, 66.8863)
  spline S129 degree 2 poles (-174.4805, 66.8863) (-175.3401, 66.8863) (-176.3182, 67.1432) (-176.664, 67.3704) knots 0 0 0 1 2 2 2
  spline S130 degree 2 poles (-176.664, 67.3704) (-177.2519, 67.7607) (-177.899, 69.05) (-177.899, 69.9392) knots 0 0 0 1 2 2 2
  spline S131 degree 2 poles (-177.0543, 69.9293) (-177.0543, 69.2278) (-176.5899, 68.2349) (-176.1305, 67.9533) knots 0 0 0 1 2 2 2
  spline S132 degree 2 poles (-176.1305, 67.9533) (-175.8045, 67.7607) (-175.0684, 67.5878) (-174.5201, 67.5878) knots 0 0 0 1 2 2 2
  line L181 (-174.5201, 67.5878) -> (-173.9025, 67.5878)
  line L182 (-173.9025, 67.5878) -> (-173.9025, 72.2808)
  line L183 (-173.9025, 72.2808) -> (-174.5201, 72.2808)
  spline S133 degree 2 poles (-174.5201, 72.2808) (-175.0585, 72.2808) (-175.8736, 72.1079) (-176.2046, 71.8757) knots 0 0 0 1 2 2 2
  spline S134 degree 2 poles (-176.2046, 71.8757) (-176.6294, 71.5892) (-177.0543, 70.6407) (-177.0543, 69.9293) knots 0 0 0 1 2 2 2
  line L184 (-178.7784, 72.9823) -> (-178.7784, 66.8863)
  line L185 (-178.7784, 66.8863) -> (-182.5921, 66.8863)
  line L186 (-182.5921, 66.8863) -> (-182.5921, 67.6075)
  line L187 (-182.5921, 67.6075) -> (-179.5885, 67.6075)
  line L188 (-179.5885, 67.6075) -> (-179.5885, 69.2772)
  line L189 (-179.5885, 69.2772) -> (-182.3895, 69.2772)
  line L190 (-182.3895, 69.2772) -> (-182.3895, 69.9985)
  line L191 (-182.3895, 69.9985) -> (-179.5885, 69.9985)
  line L192 (-179.5885, 69.9985) -> (-179.5885, 72.261)
  line L193 (-179.5885, 72.261) -> (-182.5921, 72.261)
  line L194 (-182.5921, 72.261) -> (-182.5921, 72.9823)
  line L195 (-182.5921, 72.9823) -> (-178.7784, 72.9823)
  point P0 (0, 0)
  point P1 (-30.4746, 3.2233)
  point P2 (-96.9423, 48.4423)
  point P3 (-163.3926, 66.7776)
  point P4 (-95.9828, 37.469)
  constraints: 4 other
emboss "Emboss1" sketch "Sketch6" operation cut depth 0.508 direction (0, 0, 1)
sketch "Sketch7" plane through (0, 0, 0) normal (0, 0, -1) x (-1, 0, 0)
  arc A0 (-46, 88) -> (-50, 88) centre (-48, 88) ccw construction
  circle A1 centre (-48, 88) radius 2.2
  point P0 (0, 0)
  dimension "d67" = 4.4
  constraints: 1 centre point, 1 coincident
  measures "d67" diameter of A1
extrude "Odometry module hole" cut sketch "Sketch7" against normal through all
sketch "Sketch8" plane through (0, 0, 8) normal (0, 0, 1) x (1, 0, 0)
  circle A0 centre (48, 88) radius 2.2 construction
  circle A1 centre (48, 88) radius 4.115 construction
  line L0 (48, 92.115) -> (51.5637, 90.0575)
  line L1 (51.5637, 90.0575) -> (51.5637, 85.9425)
  line L2 (51.5637, 85.9425) -> (48, 83.885)
  line L3 (48, 83.885) -> (44.4363, 85.9425)
  line L4 (44.4363, 85.9425) -> (44.4363, 90.0575)
  line L5 (44.4363, 90.0575) -> (48, 92.115)
  point P0 (0, 0)
  dimension "d70" = 8.23
  constraints: 12 end point, 2 coincident, 1 vertical alignment, 15 other
extrude "Odometry module nut well" cut sketch "Sketch8" against normal blind 6
equation "\"d26\" = SixClearanceHole"
equation "\"d27\" = SixClearanceHole"
equation "\"d28\" = SixClearanceHole"
equation "\"d29\" = SixClearanceHole"
equation "\"d30\" = SixClearanceHole"
equation "\"d31\" = SixClearanceHole"
equation "\"d32\" = SixClearanceHole"
equation "\"d33\" = SixClearanceHole"
equation "\"d34\" = SixClearanceHole"
equation "\"d35\" = SixClearanceHole"
equation "\"d36\" = SixClearanceHole"
equation "\"d37\" = SixClearanceHole"
equation "\"d38\" = SixClearanceHole"
equation "\"d39\" = SixClearanceHole"
equation "\"d40\" = SixClearanceHole"
equation "\"d42\" = SixClearanceHole"
equation "\"d49\" = SixNutWell"
equation "\"d50\" = SixNutWell"
equation "\"d51\" = SixNutWell"
equation "\"d52\" = SixNutWell"
equation "\"d53\" = SixNutWell"
equation "\"d73\" = SixNutWell"
equation "\"d74\" = SixNutWell"
equation "\"d76\" = SixNutWell"
equation "\"d77\" = SixNutWell"
equation "\"d78\" = SixNutWell"
equation "\"d79\" = SixNutWell"
equation "\"d80\" = SixNutWell"
equation "\"d81\" = SixNutWell"
body "Solid1"
